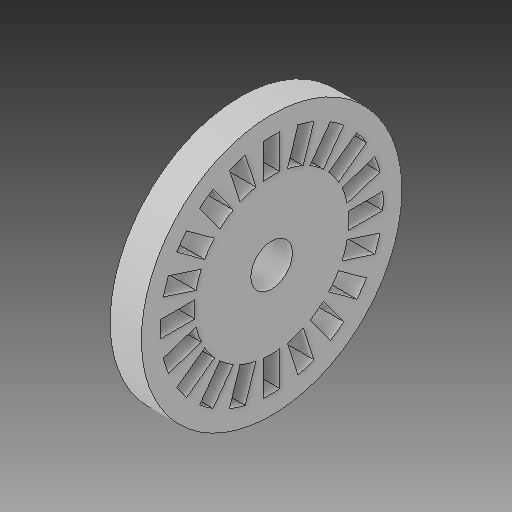
# Autodesk Inventor part: Enc_
Saved by Autodesk Inventor 2019 (Build 230136000, 136)
## iProperties
Created: 2020-01-27
Part Number: Enc_
Material: Generic
Document SubType Name: Modeling
Designer: peter
Density: 1 g/cm^3
Appearance: Default
Mass: 1.11769 g
Surface Area: 16.0834 cm^2
Volume: 1.11769 cm^3
Author: peter
Autodesk Inventor part; units mm, degrees
ref_plane "YZ Plane" through (0, 0, 0) normal (1, 0, 0) x (0, 1, 0)
ref_plane "XZ Plane" through (0, 0, 0) normal (0, 1, 0) x (-1, 0, 0)
ref_plane "XY Plane" through (0, 0, 0) normal (0, 0, 1) x (1, 0, 0)
sketch "Sketch1" plane through (0, 0, 0) normal (1, 0, 0) x (0, 1, 0)
  circle A0 centre (2.2464, -2.4677) radius 12.5
  circle A1 centre (2.2464, -2.4677) radius 2
  arc A2 (9.603, -3.2677) -> (9.603, -1.6677) centre (2.2464, -2.4677) ccw
  arc A3 (12.9165, -3.2677) -> (12.9165, -1.6677) centre (2.2464, -2.4677) ccw
  line L0 (9.603, -3.2677) -> (12.9165, -3.2677)
  line L1 (9.603, -1.6677) -> (12.9165, -1.6677)
  line L2 (8.9958, 0.5665) -> (12.147, 1.5904)
  arc A4 (12.6414, 0.0687) -> (12.147, 1.5904) centre (2.2464, -2.4677) ccw
  line L3 (9.4902, -0.9552) -> (12.6414, 0.0687)
  arc A5 (9.4902, -0.9552) -> (8.9958, 0.5665) centre (2.2464, -2.4677) ccw
  line L4 (7.7278, 2.5037) -> (10.4084, 4.4513)
  arc A6 (11.3489, 3.1568) -> (10.4084, 4.4513) centre (2.2464, -2.4677) ccw
  line L5 (8.6683, 1.2092) -> (11.3489, 3.1568)
  arc A7 (8.6683, 1.2092) -> (7.7278, 2.5037) centre (2.2464, -2.4677) ccw
  line L6 (5.9233, 3.9542) -> (7.8709, 6.6348)
  arc A8 (9.1653, 5.6944) -> (7.8709, 6.6348) centre (2.2464, -2.4677) ccw
  line L7 (7.2177, 3.0138) -> (9.1653, 5.6944)
  arc A9 (7.2177, 3.0138) -> (5.9233, 3.9542) centre (2.2464, -2.4677) ccw
  line L8 (3.7589, 4.7761) -> (4.7828, 7.9274)
  arc A10 (6.3045, 7.433) -> (4.7828, 7.9274) centre (2.2464, -2.4677) ccw
  line L9 (5.2806, 4.2817) -> (6.3045, 7.433)
  arc A11 (5.2806, 4.2817) -> (3.7589, 4.7761) centre (2.2464, -2.4677) ccw
  line L10 (1.4464, 4.889) -> (1.4464, 8.2024)
  arc A12 (3.0464, 8.2024) -> (1.4464, 8.2024) centre (2.2464, -2.4677) ccw
  line L11 (3.0464, 4.889) -> (3.0464, 8.2024)
  arc A13 (3.0464, 4.889) -> (1.4464, 4.889) centre (2.2464, -2.4677) ccw
  line L12 (-0.7878, 4.2817) -> (-1.8117, 7.433)
  arc A14 (-0.29, 7.9274) -> (-1.8117, 7.433) centre (2.2464, -2.4677) ccw
  line L13 (0.7339, 4.7761) -> (-0.29, 7.9274)
  arc A15 (0.7339, 4.7761) -> (-0.7878, 4.2817) centre (2.2464, -2.4677) ccw
  line L14 (-2.7249, 3.0138) -> (-4.6725, 5.6944)
  arc A16 (-3.3781, 6.6348) -> (-4.6725, 5.6944) centre (2.2464, -2.4677) ccw
  line L15 (-1.4305, 3.9542) -> (-3.3781, 6.6348)
  arc A17 (-1.4305, 3.9542) -> (-2.7249, 3.0138) centre (2.2464, -2.4677) ccw
  line L16 (-4.1755, 1.2092) -> (-6.8561, 3.1568)
  arc A18 (-5.9156, 4.4513) -> (-6.8561, 3.1568) centre (2.2464, -2.4677) ccw
  line L17 (-3.235, 2.5037) -> (-5.9156, 4.4513)
  arc A19 (-3.235, 2.5037) -> (-4.1755, 1.2092) centre (2.2464, -2.4677) ccw
  line L18 (-4.9974, -0.9552) -> (-8.1486, 0.0687)
  arc A20 (-7.6542, 1.5904) -> (-8.1486, 0.0687) centre (2.2464, -2.4677) ccw
  line L19 (-4.503, 0.5665) -> (-7.6542, 1.5904)
  arc A21 (-4.503, 0.5665) -> (-4.9974, -0.9552) centre (2.2464, -2.4677) ccw
  line L20 (-5.1102, -3.2677) -> (-8.4237, -3.2677)
  arc A22 (-8.4237, -1.6677) -> (-8.4237, -3.2677) centre (2.2464, -2.4677) ccw
  line L21 (-5.1102, -1.6677) -> (-8.4237, -1.6677)
  arc A23 (-5.1102, -1.6677) -> (-5.1102, -3.2677) centre (2.2464, -2.4677) ccw
  line L22 (-4.503, -5.5018) -> (-7.6542, -6.5257)
  arc A24 (-8.1486, -5.004) -> (-7.6542, -6.5257) centre (2.2464, -2.4677) ccw
  line L23 (-4.9974, -3.9801) -> (-8.1486, -5.004)
  arc A25 (-4.9974, -3.9801) -> (-4.503, -5.5018) centre (2.2464, -2.4677) ccw
  line L24 (-3.235, -7.439) -> (-5.9156, -9.3866)
  arc A26 (-6.8561, -8.0921) -> (-5.9156, -9.3866) centre (2.2464, -2.4677) ccw
  line L25 (-4.1755, -6.1446) -> (-6.8561, -8.0921)
  arc A27 (-4.1755, -6.1446) -> (-3.235, -7.439) centre (2.2464, -2.4677) ccw
  line L26 (-1.4305, -8.8895) -> (-3.3781, -11.5701)
  arc A28 (-4.6725, -10.6297) -> (-3.3781, -11.5701) centre (2.2464, -2.4677) ccw
  line L27 (-2.7249, -7.9491) -> (-4.6725, -10.6297)
  arc A29 (-2.7249, -7.9491) -> (-1.4305, -8.8895) centre (2.2464, -2.4677) ccw
  line L28 (0.7339, -9.7114) -> (-0.29, -12.8627)
  arc A30 (-1.8117, -12.3683) -> (-0.29, -12.8627) centre (2.2464, -2.4677) ccw
  line L29 (-0.7878, -9.217) -> (-1.8117, -12.3683)
  arc A31 (-0.7878, -9.217) -> (0.7339, -9.7114) centre (2.2464, -2.4677) ccw
  line L30 (3.0464, -9.8243) -> (3.0464, -13.1377)
  arc A32 (1.4464, -13.1377) -> (3.0464, -13.1377) centre (2.2464, -2.4677) ccw
  line L31 (1.4464, -9.8243) -> (1.4464, -13.1377)
  arc A33 (1.4464, -9.8243) -> (3.0464, -9.8243) centre (2.2464, -2.4677) ccw
  line L32 (5.2806, -9.217) -> (6.3045, -12.3683)
  arc A34 (4.7828, -12.8627) -> (6.3045, -12.3683) centre (2.2464, -2.4677) ccw
  line L33 (3.7589, -9.7114) -> (4.7828, -12.8627)
  arc A35 (3.7589, -9.7114) -> (5.2806, -9.217) centre (2.2464, -2.4677) ccw
  line L34 (7.2177, -7.9491) -> (9.1653, -10.6297)
  arc A36 (7.8709, -11.5701) -> (9.1653, -10.6297) centre (2.2464, -2.4677) ccw
  line L35 (5.9233, -8.8895) -> (7.8709, -11.5701)
  arc A37 (5.9233, -8.8895) -> (7.2177, -7.9491) centre (2.2464, -2.4677) ccw
  line L36 (8.6683, -6.1446) -> (11.3489, -8.0921)
  arc A38 (10.4084, -9.3866) -> (11.3489, -8.0921) centre (2.2464, -2.4677) ccw
  line L37 (7.7278, -7.439) -> (10.4084, -9.3866)
  arc A39 (7.7278, -7.439) -> (8.6683, -6.1446) centre (2.2464, -2.4677) ccw
  line L38 (9.4902, -3.9801) -> (12.6414, -5.004)
  arc A40 (12.147, -6.5257) -> (12.6414, -5.004) centre (2.2464, -2.4677) ccw
  line L39 (8.9958, -5.5018) -> (12.147, -6.5257)
  arc A41 (8.9958, -5.5018) -> (9.4902, -3.9801) centre (2.2464, -2.4677) ccw
  point P0 (0, 0)
  dimension "d7" = 5.4
  dimension "d12" = 360
  constraints: 80 end point, 80 point on circle, 42 centre point, 22 coincident, 199 other
  measures "d7" radial gap between concentric circles of A2 A1
extrude "Extrusion1" add sketch "Sketch1" along normal blind 3
body "Solid1"
